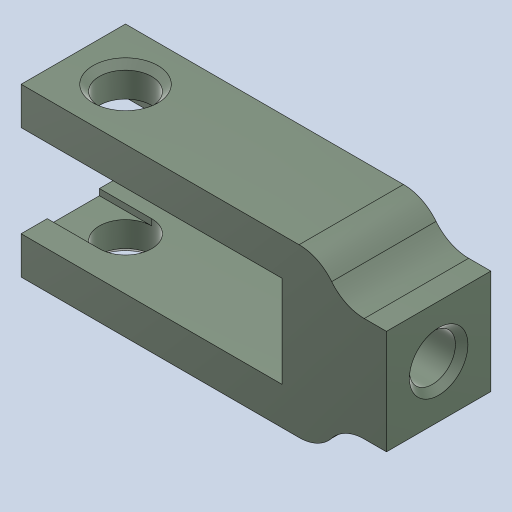
# Autodesk Inventor part: gear_1
Saved by Autodesk Inventor 2023 (Build 270158000, 158)
## iProperties
Created: 2022-06-15
Part Number: gear_1
Material: ABS プラスチック
Document SubType Name: Modeling
Designer: legot
Density: 1.06 g/cm^3
Appearance: 滑らか - 白
Author: legot
Autodesk Inventor part; units mm, degrees
ref_plane "YZ Plane" through (0, 0, 0) normal (1, 0, 0) x (0, 1, 0)
ref_plane "XZ Plane" through (0, 0, 0) normal (0, 1, 0) x (-1, 0, 0)
ref_plane "XY Plane" through (0, 0, 0) normal (0, 0, 1) x (1, 0, 0)
sketch "スケッチ1" plane through (0, 0, 0) normal (0, 1, 0) x (-1, 0, 0)
  line L0 (0, 2.5) -> (-12, 2.5)
  line L1 (-12, 2.5) -> (-12, -2.5)
  line L2 (-12, -2.5) -> (0, -2.5)
  arc A0 (0, -2.5) -> (0, 2.5) centre (0, 0) ccw
  circle A1 centre (0, 0) radius 1.25
  line L3 (0, 2.5) -> (2.5, 2.5)
  line L4 (2.5, 2.5) -> (2.5, -2.5)
  line L5 (2.5, -2.5) -> (0, -2.5)
  point P0 (2.5, 0)
  dimension "d0" = 2.5
  dimension "d1" = 2.5
  dimension "d2" = 12
  constraints: 12 end point, 3 perpendicular, 3 tangent, 2 centre point, 2 coincident, 2 horizontal, 2 point on circle, 1 parallel
  measures "d0" radius of A0
  measures "d1" diameter of A1
  measures "d2" distance from line of point (0, 0) L1
extrude "押し出し1" add sketch "スケッチ1" along normal mid plane 8
sketch "スケッチ7" plane through (-2.5, 4, 2.5) normal (0, 0, 1) x (1, 0, 0)
  line L0 (14.5, 0) -> (14.5, -8) projected
  line L1 (0, -8) -> (0, 0) projected
  line L2 (0, -8) -> (0, 0) projected
  line L3 (0, -1.8) -> (11.5, -1.8)
  line L4 (11.5, -1.8) -> (11.5, -6.2)
  line L5 (11.5, -6.2) -> (0, -6.2)
  line L6 (0, -6.2) -> (0, -1.8)
  line L7 (0, 0) -> (14.5, 0) projected
  point P0 (2.5, -4)
  point P1 (0, -4)
  point P2 (0, -1.8)
  point P3 (0, -6.2)
  dimension "d32" = 3
  dimension "d46" = 4.4
  dimension "d47" = 1.8
  constraints: 8 end point, 2 midpoint, 2 parallel, 1 horizontal, 1 perpendicular, 1 point on line
  measures "d32" distance between parallel lines of L0 L4
  measures "d46" distance between parallel lines of L5 L3
  measures "d47" distance between parallel lines of L7 L3
extrude "押し出し5" cut sketch "スケッチ7" against normal through all
sketch "スケッチ3" plane through (12, -4, 2.5) normal (1, 0, 0) x (0, 0, -1)
  line L0 (5, 0) -> (5, 8) projected
  line L1 (0, 8) -> (0, 0) projected
  line L2 (0, 6.5) -> (5, 6.5)
  line L3 (5, 6.5) -> (5, 1.5)
  line L4 (5, 1.5) -> (0, 1.5)
  line L5 (0, 1.5) -> (0, 6.5)
  point P0 (2.5, 4)
  point P1 (0, 4)
  point P2 (0, 4)
  point P3 (0, 6.5)
  constraints: 8 end point, 2 collinear, 2 midpoint, 2 parallel, 2 perpendicular, 1 coincident, 1 horizontal
extrude "押し出し3" add sketch "スケッチ3" along normal blind 3
sketch "スケッチ5" plane through (0, 0, 0) normal (0, 1, 0) x (-1, 0, 0)
  line L0 (6.0321, 1.25) -> (0, 1.25)
  line L1 (0, 1.25) -> (0, -1.25)
  line L2 (0, -1.25) -> (6.0321, -1.25)
  line L3 (6.0321, -1.25) -> (6.0321, 1.25)
  circle A0 centre (0, 0) radius 1.25 projected
  constraints: 8 end point, 2 parallel, 2 tangent, 1 horizontal, 1 midpoint, 1 perpendicular
extrude "押し出し4" cut sketch "スケッチ5" along normal mid plane 5 contours L3 L2 A0 L0 | A0 L1 picked at (0.2598, 0.3258)
sketch "スケッチ8" plane through (15, -4, 2.5) normal (1, 0, 0) x (0, 0, -1)
  point P0 (2.5, 4)
  point P1 (2.5, 4)
  constraints: 1 coincident
hole "穴3" at (15, 0, 0) direction (-1, 0, 0) diameter 2.2 end through all
fillet "フィレット2" radius 2 4 edges at (12, 4, 0) (12, -4, 0) (12, -2.5, 0) (12, 2.5, 0)
chamfer "面取り1" distance 0.3 angle 45 3 edges at (1.25, 4, 0) (1.25, -4, 0) (15, 0, 1.1)
chamfer "面取り2" distance 1 angle 45 2 edges at (9, 0, 2.5) (9, 0, -2.5)
fillet "フィレット4" radius 1 2 edges at (9, 2.2, 0) (9, -2.2, 0)
